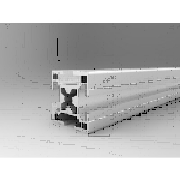
# Autodesk Inventor part: perfil_estrutural_30x30-01
Saved by Autodesk Inventor 2018 (Build 220112000, 112)
## iProperties
Created: 2018-08-20
Part Number: perfil_estrutural_30x30-01
Material: Alumínio 6061
Description: Perfil Estrutural em Alumínio 30x30 Parafuso - centro M8, Código do produto: PF30-11
Document SubType Name: Modeling
Standard: Sem nome
Designer: Georgines
Manufacturer: https://loja.forsetisolucoes.com.br
Language: pt-BR
Size Designation: 30 x30 xperfil_estrutural_30x30-01
Categories: <MemberInstance><Categories><Category DisplayName="Formas estruturais" InternalName="089c4875-fa83-4c05-b084-43b9cc11f5ed" Mnemonic="GRDR"><CategoryParameter DisplayName="Massa por unidade de comprimento" InternalName="0bb95a10-148f-4027-a459-38d7b056702a" Mnemonic="shpmass"/><CategoryParameter DisplayName="Área do perfil" InternalName="1ff91680-64b0-4202-b9a3-7fd3f94bba3b" Mnemonic="secarea"/><CategoryParameter DisplayName="Raio de rotação (x)" InternalName="25778675-03e9-40c1-b6a8-4a9ed693320d" Mnemonic="gyrradx"/><CategoryParameter DisplayName="Módulo de torção" InternalName="26c1ec35-5026-4c63-ad0a-751cf684a536" Mnemonic="torrigmod"/><CategoryParameter DisplayName="Distância do centro de gravidade X-X" InternalName="26c9bdb8-9c79-4b4f-a92e-8e197583c9c4" Mnemonic="grcendistX"/><CategoryParameter DisplayName="ID de membro antiga" InternalName="340afe4f-75d7-48d3-ab7d-943f3c3da468" Mnemonic="LegacyMemberID"/><CategoryParameter DisplayName="Comprimento da base" InternalName="42e34263-8f20-4d0e-ad48-bf1385b87c24" Mnemonic="shplen"/><CategoryParameter DisplayName="Momento de inércia (y)" InternalName="4b9f58ea-bced-460e-81ea-3d29ca5a49e3" Mnemonic="inermomy"/><CategoryParameter DisplayName="Momento de inércia (x)" InternalName="4cd780bc-73d7-43ac-917a-579e5cbd684d" Mnemonic="inermomx"/><CategoryParameter DisplayName="Ponto base customizado" InternalName="4f1d1b73-316d-484b-a3df-9cbabb16eb77" Mnemonic="shpBasePoint"/><CategoryParameter DisplayName="Altura da forma" InternalName="50274e7d-5ac0-4796-92cb-c59e54983c67" Mnemonic="shpheig"/><CategoryParameter DisplayName="Módulo do perfil (y)" InternalName="59eaa5e9-d227-48dc-b6c1-6920f96e0f95" Mnemonic="secmody"/><CategoryParameter DisplayName="Designação do perfil" InternalName="5a64d034-428d-49c8-ba32-7619764de20f" Mnemonic="shpdes"/><CategoryParameter DisplayName="Módulo do perfil (x)" InternalName="72cfad18-cf51-4ed4-aaa7-c6b224f8419f" Mnemonic="secmodx"/><CategoryParameter DisplayName="Módulo de torção do perfil" InternalName="7c55a8dc-8844-49f9-a867-cc677b30ec9a" Mnemonic="torsecmod"/><CategoryParameter DisplayName="Largura da forma" InternalName="7c717d54-a18f-4666-b4d4-573cce22c62c" Mnemonic="shpwdth"/><CategoryParameter DisplayName="Espessura da segunda forma" InternalName="9251a8e1-85fd-4e47-af99-afdb762317d9" Mnemonic="shpthick2"/><CategoryParameter DisplayName="Iniciado por FG" InternalName="9c666724-f362-4ea7-ac62-f6a007de5c69" Mnemonic="shpFGAuto"/><CategoryParameter DisplayName="Distância do centro de gravidade Y-Y" InternalName="bcc4fb17-7af4-436a-8f8c-d0aa3b0248c5" Mnemonic="grcendistY"/><CategoryParameter DisplayName="Raio de rotação (y)" InternalName="bfa18ebe-1636-4dbe-8d42-b263e0b73184" Mnemonic="gyrrady"/><CategoryParameter DisplayName="Espessura da forma" InternalName="d109cf76-8eb4-42fc-9800-4409734adc67" Mnemonic="shpthick"/><CategoryParameter DisplayName="Coeficiente de deslocamento por cisalhamento" InternalName="de4c90c6-aaa8-468f-a335-6737b311b5d3" Mnemonic="shdispc"/><Category DisplayName="Outro" InternalName="f02205ff-2390-476f-921c-0b3185f88e84" Mnemonic="OTHSHP"><CategoryParameter DisplayName="Momento de inércia (y)" InternalName="044c654e-f649-48ac-84cc-650a29ae31ca" Mnemonic="inermomy"/><CategoryParameter DisplayName="Espessura da forma" InternalName="12b1a788-9233-48fd-a933-2df8ff42b15f" Mnemonic="shpthick"/><CategoryParameter DisplayName="Massa por unidade de comprimento" InternalName="2fd289d6-9394-4d2d-97e6-6659d7d4551d" Mnemonic="shpmass"/><CategoryParameter DisplayName="Raio de rotação (y)" InternalName="743e1dfe-1bba-408b-b985-cf752b207386" Mnemonic="gyrrady"/><CategoryParameter DisplayName="Módulo do perfil (y)" InternalName="88b8bff9-a616-4028-93d5-ed4f79680d13" Mnemonic="secmody"/><CategoryParameter DisplayName="Área do perfil" InternalName="c46ecdf8-b6eb-4db9-8b25-30258930c1e3" Mnemonic="secarea"/><CategoryParameter DisplayName="Módulo do perfil (x)" InternalName="cac70804-9d39-43bb-be17-56ea1f39a6c2" Mnemonic="secmodx"/><CategoryParameter DisplayName="Momento de inércia (x)" InternalName="ec6737bc-264f-43ed-b0bd-f6d410c2718d" Mnemonic="inermomx"/><CategoryParameter DisplayName="Raio de rotação (x)" InternalName="ee72c61e-565e-4fd6-b448-66e1e1abcb7e" Mnemonic="gyrradx"/></Category></Category><Category DisplayName="Tipo de dado" InternalName="23b78d0f-2648-40c6-8793-ca6db495c9e8" Mnemonic="DATATYPE"><CategoryParameter DisplayName="Nome de exibição" InternalName="05415f3d-3907-474b-a020-eb9d644f4cf3" Mnemonic="DISPLAYNAME"/><CategoryParameter DisplayName="Padrão" InternalName="0c0a119c-1e12-4c84-803f-101930972f5e" Mnemonic="STANDARD"/><CategoryParameter DisplayName="Descrição" InternalName="13903e3d-64b1-4950-80da-f627842ea37f" Mnemonic="DESCRIPTION"/><CategoryParameter DisplayName="Designação" InternalName="2675968c-4ce5-49e0-a4f5-552d29089031" Mnemonic="DESIGNATION"/><CategoryParameter DisplayName="Fileira padrão" InternalName="2af9ec52-faaa-4026-b378-f9fa4afca842" Mnemonic="DEFAULTROW"/><CategoryParameter DisplayName="Nome da pasta" InternalName="3f06958e-8713-4116-9be7-ed6184ecc97b" Mnemonic="FOLDERNAME"/><CategoryParameter DisplayName="Guia de revisão" InternalName="45a75005-10b1-4dfc-8d6d-dfe629f0b93c" Mnemonic="REVISIONGUID"/><CategoryParameter DisplayName="Nome do arquivo" InternalName="8b46a4cc-9585-4fed-90c3-899f57e09a73" Mnemonic="FILENAME"/><CategoryParameter DisplayName="OrgPad" InternalName="8f5914e1-4693-403f-8ab5-d37768198c9d" Mnemonic="STDSORG"/><CategoryParameter DisplayName="Versão da família" InternalName="914462f6-6e19-4b14-ba84-155b9680b1d0" Mnemonic="FAMILYREVISION"/><CategoryParameter DisplayName="Revisão padrão" InternalName="91d5a463-65c2-4fde-b823-3b7fea5e8e17" Mnemonic="STANDARDREVISION"/><CategoryParameter DisplayName="Revisão do membro" InternalName="a65d44b9-392f-4f4f-857b-e4b3d54996fe" Mnemonic="MEMBERREVISION"/><CategoryParameter DisplayName="Formato do anel" InternalName="bc51e27b-3422-4e78-93ef-cec197ddf230" Mnemonic="CLIPFORMAT"/><CategoryParameter DisplayName="Fabricante" InternalName="cd6c7a72-a28a-4e50-99a9-2c7f4e13e5ad" Mnemonic="MANUFACTURER"/><CategoryParameter DisplayName="Nome interno" InternalName="cf1d0246-76d9-4b4a-8305-fa0409afb5c1" Mnemonic="INTERNALNAME"/><CategoryParameter DisplayName="Métrico" InternalName="e2385c5b-1ea4-4823-96a8-8de651266ec3" Mnemonic="ISMETRIC"/><Category DisplayName="Peça" InternalName="c0e0b642-3bcb-4cc8-9e80-f96d35c4afa4" Mnemonic="PART"><CategoryParameter DisplayName="Núm. de peça" InternalName="016b6077-bfbe-49bd-92c9-d8d59c39c941" Mnemonic="PARTNUMBER"/><CategoryParameter DisplayName="Núm. de estoque" InternalName="4dba7c1c-e26c-444e-836c-b08b433409a8" Mnemonic="STOCKNUMBER"/><CategoryParameter DisplayName="Chaveta de material" InternalName="5c9a8adb-dd2b-4535-b97f-0a94a95fe41f" Mnemonic="MATERIALKEY"/><CategoryParameter DisplayName="Material" InternalName="818a152a-d3c3-49ca-80ee-df7d91421b8e" Mnemonic="MATERIAL"/></Category></Category></Categories><FamilyTemplate Id="perfil_estrutural_30x30"><FamilyTemplateParameters><FamilyTemplateParameter ObjectType="kUserParameterObject" ValueType="xs:double" Id="1" ObjectReferenceKey="ALTURA"/><FamilyTemplateParameter ObjectType="kUserParameterObject" ValueType="xs:double" Id="2" ObjectReferenceKey="COMPRIMENTO"/><FamilyTemplateParameter ObjectType="kUserParameterObject" ValueType="xs:double" Id="3" ObjectReferenceKey="LARGURA"/><FamilyTemplateParameter ObjectType="kPartComponentDefinitionObject" ValueType="xs:string" Id="6" SubObjectId="Material"/><FamilyTemplateParameter ObjectType="kPropertyObject" ValueType="xs:string" Id="18" ObjectReferenceKey="{32853F0F-3444-11d1-9E93-0060B03C1CA6}" SubObjectId="5"/><FamilyTemplateParameter ObjectType="kPropertyObject" ValueType="xs:string" Id="19" ObjectReferenceKey="{32853F0F-3444-11d1-9E93-0060B03C1CA6}" SubObjectId="52"/></FamilyTemplateParameters></FamilyTemplate><CategoryParameterMap><ParamToTemplateMap><ParamToTemplate CategoryParameter="//CategoryParameter[@InternalName='cf1d0246-76d9-4b4a-8305-fa0409afb5c1']" ConstantValue="80671f61-67d6-4e80-bcd6-88f6d3e07490"/><ParamToTemplate CategoryParameter="//CategoryParameter[@InternalName='45a75005-10b1-4dfc-8d6d-dfe629f0b93c']" ConstantValue="1a1e662f-2d83-4367-9875-4263c100c1bc"/><ParamToTemplate CategoryParameter="//CategoryParameter[@InternalName='3f06958e-8713-4116-9be7-ed6184ecc97b']" ConstantValue="Perfil strutural 30 x 30 - centro m8"/><ParamToTemplate CategoryParameter="//CategoryParameter[@InternalName='8f5914e1-4693-403f-8ab5-d37768198c9d']" TemplateParameter="11"/><ParamToTemplate CategoryParameter="//CategoryParameter[@InternalName='0c0a119c-1e12-4c84-803f-101930972f5e']" TemplateParameter="12"/><ParamToTemplate CategoryParameter="//CategoryParameter[@InternalName='91d5a463-65c2-4fde-b823-3b7fea5e8e17']" TemplateParameter="13"/><ParamToTemplate CategoryParameter="//CategoryParameter[@InternalName='cd6c7a72-a28a-4e50-99a9-2c7f4e13e5ad']" ConstantValue="https://loja.forsetisolucoes.com.br"/><ParamToTemplate CategoryParameter="//CategoryParameter[@InternalName='13903e3d-64b1-4950-80da-f627842ea37f']" ConstantValue="Perfil Estrutural em Alumínio 30x30 Parafuso - centro M8, Código do produto: PF30-11"/><ParamToTemplate CategoryParameter="//CategoryParameter[@InternalName='05415f3d-3907-474b-a020-eb9d644f4cf3']" ConstantValue="Perfil strutural 30 x 30 - centro m8"/><ParamToTemplate CategoryParameter="//CategoryParameter[@InternalName='914462f6-6e19-4b14-ba84-155b9680b1d0']" ConstantValue="11"/><ParamToTemplate CategoryParameter="//CategoryParameter[@InternalName='bc51e27b-3422-4e78-93ef-cec197ddf230']" ConstantValue="CF_INVENTOR.STDPARTS"/><ParamToTemplate CategoryParameter="//CategoryParameter[@InternalName='e2385c5b-1ea4-4823-96a8-8de651266ec3']" ConstantValue="true"/><ParamToTemplate CategoryParameter="//CategoryParameter[@InternalName='2af9ec52-faaa-4026-b378-f9fa4afca842']" ConstantValue="1"/><ParamToTemplate CategoryParameter="//CategoryParameter[@InternalName='9c666724-f362-4ea7-ac62-f6a007de5c69']" ConstantValue="1"/><ParamToTemplate CategoryParameter="//CategoryParameter[@InternalName='8b46a4cc-9585-4fed-90c3-899f57e09a73']" ConstantValue="perfil_estrutural_30x30-01"/><ParamToTemplate CategoryParameter="//CategoryParameter[@InternalName='a65d44b9-392f-4f4f-857b-e4b3d54996fe']" ConstantValue="2f49c4fb-9da5-4441-ae67-751848dc7a1d"/><ParamToTemplate CategoryParameter="//CategoryParameter[@InternalName='a65d44b9-392f-4f4f-857b-e4b3d54996fe']" ConstantValue="2f49c4fb-9da5-4441-ae67-751848dc7a1d"/><ParamToTemplate CategoryParameter="//CategoryParameter[@InternalName='42e34263-8f20-4d0e-ad48-bf1385b87c24']" TemplateParameter="2"/><ParamToTemplate CategoryParameter="//CategoryParameter[@InternalName='2675968c-4ce5-49e0-a4f5-552d29089031']" TemplateParameter="19"/><ParamToTemplate CategoryParameter="//CategoryParameter[@InternalName='818a152a-d3c3-49ca-80ee-df7d91421b8e']" TemplateParameter="6"/><ParamToTemplate CategoryParameter="//CategoryParameter[@InternalName='016b6077-bfbe-49bd-92c9-d8d59c39c941']" TemplateParameter="18"/></ParamToTemplateMap></CategoryParameterMap></MemberInstance>
Density: 2.7 g/cm^3
Appearance: Alumínio - Plano
_CCFamilyMember: 1
_CCFamilyDisplayName: Perfil strutural 30 x 30 - centro m8 - Perfil Estrutural em Alumínio 30x30 Parafuso - centro M8, Código do produto: PF30-11
_FrameMemberDoc: Frame Member File
_Version: 15.0.0
_GetPNFromCC: 1
IsCustomPart: 1
Author: Georgines
G_L: 490,000 mm
G_W: 30,000 mm
G_H: 30,000 mm
Autodesk Inventor part; units mm, degrees
ref_plane "YZ Plane" through (0, 0, 0) normal (1, 0, 0) x (0, 1, 0)
ref_plane "Plano inicial" through (0, 0, 0) normal (0, 0, 1) x (1, 0, 0)
ref_plane "Plano final" through (0, 0, 490) normal (0, 0, 1) x (1, 0, 0)
sketch "Esboço" plane through (0, 0, 0) normal (0, 0, 1) x (1, 0, 0)
  line L0 (15, -6.6) -> (15, -4.05)
  line L1 (15, -4.05) -> (13, -4.05)
  line L2 (15, -13.5) -> (15, -8.8)
  line L3 (15, -8.8) -> (14.7, -8.8)
  arc A0 (13.5, -15) -> (15, -13.5) centre (13.5, -13.5) ccw
  arc A1 (7.9, -6.2201) -> (7.9879, -6.4322) centre (8.2, -6.2201) ccw
  arc A2 (6.4322, -7.9879) -> (6.2201, -7.9) centre (6.2201, -8.2) ccw
  arc A3 (9, -10.6799) -> (8.9121, -10.4678) centre (8.7, -10.6799) ccw
  arc A4 (10.3, -10) -> (10, -10.3) centre (10.3, -10.3) ccw
  line L4 (10.4678, -8.9121) -> (7.9879, -6.4322)
  arc A5 (10.4678, -8.9121) -> (10.6799, -9) centre (10.6799, -8.7) ccw
  line L5 (9, -10.6799) -> (9, -12.7)
  line L6 (13, -4.05) -> (13, -8.7)
  line L7 (8.7, -13) -> (4.05, -13)
  arc A6 (8.7, -13) -> (9, -12.7) centre (8.7, -12.7) ccw
  line L8 (10, -10.3) -> (10, -12.7)
  line L9 (12.7, -9) -> (10.6799, -9)
  line L10 (12.7, -10) -> (10.3, -10)
  line L11 (4.05, -15) -> (6.6, -15)
  line L12 (4.05, -13) -> (4.05, -15)
  arc A7 (12.7, -9) -> (13, -8.7) centre (12.7, -8.7) ccw
  arc A8 (13, -10.3) -> (12.7, -10) centre (12.7, -10.3) ccw
  arc A9 (10, -12.7) -> (10.3, -13) centre (10.3, -12.7) ccw
  line L13 (14.7, -8.8) -> (14.7, -6.6)
  line L14 (14.7, -6.6) -> (15, -6.6)
  line L15 (6.6, -14.7) -> (8.8, -14.7)
  line L16 (6.6, -15) -> (6.6, -14.7)
  line L17 (8.8, -14.7) -> (8.8, -15)
  line L18 (10.3, -13) -> (12.7, -13)
  arc A10 (12.7, -13) -> (13, -12.7) centre (12.7, -12.7) ccw
  line L19 (8.8, -15) -> (13.5, -15)
  line L20 (13, -12.7) -> (13, -10.3)
  arc A11 (2.9924, -5.85) -> (3.4254, -6.1) centre (3.4254, -5.6) ccw
  line L21 (3.4254, -6.1) -> (5.6, -6.1)
  arc A12 (5.6, -6.1) -> (6.1, -5.6) centre (5.6, -5.6) ccw
  line L22 (5.85, -2.9924) -> (3.097, -1.403)
  arc A13 (-1.403, -3.097) -> (1.403, -3.097) centre (0, 0) ccw
  arc A14 (6.1, -3.4254) -> (5.85, -2.9924) centre (5.6, -3.4254) ccw
  line L23 (6.1, -5.6) -> (6.1, -3.4254)
  line L24 (1.403, -3.097) -> (2.9924, -5.85)
  line L25 (6.4322, -7.9879) -> (8.9121, -10.4678)
  line L26 (-6.2201, -7.9) -> (6.2201, -7.9)
  line L27 (-3.097, -1.403) -> (-5.85, -2.9924)
  line L28 (-2.9924, -5.85) -> (-1.403, -3.097)
  arc A15 (-5.85, -2.9924) -> (-6.1, -3.4254) centre (-5.6, -3.4254) ccw
  arc A16 (-3.4254, -6.1) -> (-2.9924, -5.85) centre (-3.4254, -5.6) ccw
  line L29 (-5.6, -6.1) -> (-3.4254, -6.1)
  arc A17 (-6.1, -5.6) -> (-5.6, -6.1) centre (-5.6, -5.6) ccw
  line L30 (-6.1, -3.4254) -> (-6.1, -5.6)
  arc A18 (13, 8.7) -> (12.7, 9) centre (12.7, 8.7) ccw
  line L31 (10.6799, 9) -> (12.7, 9)
  arc A19 (12.7, 10) -> (13, 10.3) centre (12.7, 10.3) ccw
  arc A20 (10.6799, 9) -> (10.4678, 8.9121) centre (10.6799, 8.7) ccw
  arc A21 (7.9879, 6.4322) -> (7.9, 6.2201) centre (8.2, 6.2201) ccw
  line L32 (7.9879, 6.4322) -> (10.4678, 8.9121)
  line L33 (10.3, 10) -> (12.7, 10)
  arc A22 (10, 10.3) -> (10.3, 10) centre (10.3, 10.3) ccw
  line L34 (13, 10.3) -> (13, 12.7)
  arc A23 (8.9121, 10.4678) -> (9, 10.6799) centre (8.7, 10.6799) ccw
  arc A24 (13, 12.7) -> (12.7, 13) centre (12.7, 12.7) ccw
  line L35 (15, 8.8) -> (15, 13.5)
  arc A25 (6.2201, 7.9) -> (6.4322, 7.9879) centre (6.2201, 8.2) ccw
  line L36 (8.9121, 10.4678) -> (6.4322, 7.9879)
  arc A26 (15, 13.5) -> (13.5, 15) centre (13.5, 13.5) ccw
  line L37 (12.7, 13) -> (10.3, 13)
  arc A27 (10.3, 13) -> (10, 12.7) centre (10.3, 12.7) ccw
  line L38 (13.5, 15) -> (8.8, 15)
  line L39 (9, 12.7) -> (9, 10.6799)
  arc A28 (9, 12.7) -> (8.7, 13) centre (8.7, 12.7) ccw
  line L40 (8.8, 15) -> (8.8, 14.7)
  line L41 (8.8, 14.7) -> (6.6, 14.7)
  line L42 (6.6, 14.7) -> (6.6, 15)
  line L43 (4.05, 13) -> (8.7, 13)
  line L44 (4.05, 15) -> (4.05, 13)
  line L45 (6.6, 15) -> (4.05, 15)
  line L46 (10, 12.7) -> (10, 10.3)
  line L47 (7.9, -6.2201) -> (7.9, 6.2201)
  arc A29 (3.097, -1.403) -> (3.097, 1.403) centre (0, 0) ccw
  arc A30 (-3.097, 1.403) -> (-3.097, -1.403) centre (0, 0) ccw
  line L48 (-5.85, 2.9924) -> (-3.097, 1.403)
  line L49 (3.097, 1.403) -> (5.85, 2.9924)
  arc A31 (1.403, 3.097) -> (-1.403, 3.097) centre (0, 0) ccw
  arc A32 (-6.1, 3.4254) -> (-5.85, 2.9924) centre (-5.6, 3.4254) ccw
  line L50 (-6.1, 5.6) -> (-6.1, 3.4254)
  line L51 (-3.4254, 6.1) -> (-5.6, 6.1)
  arc A33 (-5.6, 6.1) -> (-6.1, 5.6) centre (-5.6, 5.6) ccw
  line L52 (6.2201, 7.9) -> (-6.2201, 7.9)
  line L53 (-1.403, 3.097) -> (-2.9924, 5.85)
  arc A34 (-2.9924, 5.85) -> (-3.4254, 6.1) centre (-3.4254, 5.6) ccw
  line L54 (2.9924, 5.85) -> (1.403, 3.097)
  arc A35 (5.85, 2.9924) -> (6.1, 3.4254) centre (5.6, 3.4254) ccw
  arc A36 (3.4254, 6.1) -> (2.9924, 5.85) centre (3.4254, 5.6) ccw
  line L55 (5.6, 6.1) -> (3.4254, 6.1)
  arc A37 (6.1, 5.6) -> (5.6, 6.1) centre (5.6, 5.6) ccw
  line L56 (6.1, 3.4254) -> (6.1, 5.6)
  line L57 (14.7, 8.8) -> (15, 8.8)
  line L58 (14.7, 6.6) -> (14.7, 8.8)
  line L59 (15, 6.6) -> (14.7, 6.6)
  line L60 (13, 4.05) -> (15, 4.05)
  line L61 (15, 4.05) -> (15, 6.6)
  line L62 (13, 8.7) -> (13, 4.05)
  arc A38 (-10.3, -13) -> (-10, -12.7) centre (-10.3, -12.7) ccw
  line L63 (-14.7, -8.8) -> (-15, -8.8)
  line L64 (-10.6799, -9) -> (-12.7, -9)
  arc A39 (-10.6799, -9) -> (-10.4678, -8.9121) centre (-10.6799, -8.7) ccw
  arc A40 (-13, -8.7) -> (-12.7, -9) centre (-12.7, -8.7) ccw
  arc A41 (-6.2201, -7.9) -> (-6.4322, -7.9879) centre (-6.2201, -8.2) ccw
  line L65 (-10.3, -10) -> (-12.7, -10)
  arc A42 (-10, -10.3) -> (-10.3, -10) centre (-10.3, -10.3) ccw
  arc A43 (-8.9121, -10.4678) -> (-9, -10.6799) centre (-8.7, -10.6799) ccw
  line L66 (-8.9121, -10.4678) -> (-6.4322, -7.9879)
  line L67 (-10, -12.7) -> (-10, -10.3)
  line L68 (-9, -12.7) -> (-9, -10.6799)
  arc A44 (-9, -12.7) -> (-8.7, -13) centre (-8.7, -12.7) ccw
  line L69 (-13, -10.3) -> (-13, -12.7)
  line L70 (-12.7, -13) -> (-10.3, -13)
  arc A45 (-13, -12.7) -> (-12.7, -13) centre (-12.7, -12.7) ccw
  line L71 (-4.05, -13) -> (-8.7, -13)
  line L72 (-15, -8.8) -> (-15, -13.5)
  line L73 (-4.05, -15) -> (-4.05, -13)
  line L74 (-6.6, -15) -> (-4.05, -15)
  line L75 (-8.8, -14.7) -> (-6.6, -14.7)
  line L76 (-6.6, -14.7) -> (-6.6, -15)
  line L77 (-8.8, -15) -> (-8.8, -14.7)
  line L78 (-13.5, -15) -> (-8.8, -15)
  arc A46 (-15, -13.5) -> (-13.5, -15) centre (-13.5, -13.5) ccw
  arc A47 (-12.7, -10) -> (-13, -10.3) centre (-12.7, -10.3) ccw
  arc A48 (-12.7, 9) -> (-13, 8.7) centre (-12.7, 8.7) ccw
  line L79 (-12.7, 9) -> (-10.6799, 9)
  arc A49 (-13, 10.3) -> (-12.7, 10) centre (-12.7, 10.3) ccw
  arc A50 (-10.4678, 8.9121) -> (-10.6799, 9) centre (-10.6799, 8.7) ccw
  arc A51 (-7.9, 6.2201) -> (-7.9879, 6.4322) centre (-8.2, 6.2201) ccw
  line L80 (-10.4678, 8.9121) -> (-7.9879, 6.4322)
  line L81 (-12.7, 10) -> (-10.3, 10)
  arc A52 (-10.3, 10) -> (-10, 10.3) centre (-10.3, 10.3) ccw
  line L82 (-13, 12.7) -> (-13, 10.3)
  arc A53 (-9, 10.6799) -> (-8.9121, 10.4678) centre (-8.7, 10.6799) ccw
  line L83 (-15, 13.5) -> (-15, 8.8)
  arc A54 (-6.4322, 7.9879) -> (-6.2201, 7.9) centre (-6.2201, 8.2) ccw
  line L84 (-6.4322, 7.9879) -> (-8.9121, 10.4678)
  arc A55 (-13.5, 15) -> (-15, 13.5) centre (-13.5, 13.5) ccw
  line L85 (-10, 10.3) -> (-10, 12.7)
  line L86 (-9, 10.6799) -> (-9, 12.7)
  line L87 (-10.3, 13) -> (-12.7, 13)
  arc A56 (-10, 12.7) -> (-10.3, 13) centre (-10.3, 12.7) ccw
  arc A57 (-8.7, 13) -> (-9, 12.7) centre (-8.7, 12.7) ccw
  line L88 (-8.8, 15) -> (-13.5, 15)
  line L89 (-8.8, 14.7) -> (-8.8, 15)
  line L90 (-6.6, 14.7) -> (-8.8, 14.7)
  line L91 (-6.6, 15) -> (-6.6, 14.7)
  line L92 (-8.7, 13) -> (-4.05, 13)
  line L93 (-4.05, 13) -> (-4.05, 15)
  line L94 (-4.05, 15) -> (-6.6, 15)
  arc A58 (-12.7, 13) -> (-13, 12.7) centre (-12.7, 12.7) ccw
  line L95 (-14.7, 8.8) -> (-14.7, 6.6)
  line L96 (-14.7, 6.6) -> (-15, 6.6)
  line L97 (-13, 4.05) -> (-13, 8.7)
  line L98 (-15, 4.05) -> (-13, 4.05)
  line L99 (-15, 6.6) -> (-15, 4.05)
  line L100 (-15, 8.8) -> (-14.7, 8.8)
  line L101 (-14.7, -6.6) -> (-14.7, -8.8)
  line L102 (-15, -6.6) -> (-14.7, -6.6)
  arc A59 (-7.9879, -6.4322) -> (-7.9, -6.2201) centre (-8.2, -6.2201) ccw
  line L103 (-13, -4.05) -> (-15, -4.05)
  line L104 (-15, -4.05) -> (-15, -6.6)
  line L105 (-13, -8.7) -> (-13, -4.05)
  line L106 (-7.9, 6.2201) -> (-7.9, -6.2201)
  line L107 (-7.9879, -6.4322) -> (-10.4678, -8.9121)
  point P0 (0, 0)
  dimension "ALTURA" = 30
  dimension "LARGURA" = 30
  constraints: 216 end point, 120 point on circle, 60 centre point
  measures "ALTURA" distance between parallel lines of L78 L88
  measures "LARGURA" distance between parallel lines of L35 L83
extrude "Corpo" add sketch "Esboço" along normal up to surface (490 mm away) from surface at 0
sketch "Esboço2" plane through (0, 0, 0) normal (0, 0, 1) x (1, 0, 0)
  line L0 (0, 0) -> (10, 0)
ref_plane "Plano de trabalho3" through (0, 0, 0) normal (0, -1, 0) x (1, 0, 0)
sketch "Esboço3" plane through (0, 0, 0) normal (0, -1, 0) x (1, 0, 0)
  line L0 (-2, 0) -> (12, 0)
  line L1 (-2, 490) -> (12, 490)
  dimension "d10" = 490
  measures "d10" distance between parallel lines of L0 L1
equation "\"G_OFFSET_START\" = 0"
equation "\"G_OFFSET_END\" = 0"
equation "\"G_L\" = d10"
